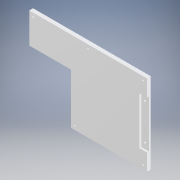
# Autodesk Inventor part: SP001b
Saved by Autodesk Inventor 2017 SP1 (Build 210196100, 196)
## iProperties
Created: 2018-01-11
Part Number: SP001b
Material: ABS Plastic
Document SubType Name: Modeling
Designer: Zach
Density: 1.06 g/cm^3
Appearance: CR White
Author: Zach
Autodesk Inventor part; units mm, degrees
ref_plane "YZ Plane" through (0, 0, 0) normal (1, 0, 0) x (0, 1, 0)
ref_plane "XZ Plane" through (0, 0, 0) normal (0, 1, 0) x (-1, 0, 0)
ref_plane "XY Plane" through (0, 0, 0) normal (0, 0, 1) x (1, 0, 0)
sketch "Sketch1" plane through (0, 0, 0) normal (0, 0, 1) x (1, 0, 0)
  line L0 (0, 0) -> (620, 0)
  line L1 (110, -213) -> (510, -213)
  line L2 (510, -213) -> (510, -80)
  line L3 (510, -80) -> (620, -80)
  line L4 (620, -80) -> (620, 0)
  line L5 (110, -213) -> (110, -80)
  line L6 (0, -80) -> (0, 0)
  line L7 (0, -80) -> (110, -80)
  point P0 (310, -213)
  point P1 (310, 0)
  dimension "d0" = 620
  dimension "d1" = 213
  dimension "d2" = 400
  dimension "d3" = 133
  constraints: 16 end point, 3 perpendicular, 2 horizontal, 2 midpoint, 2 parallel, 2 point on line, 1 vertical, 1 vertical alignment
  measures "d0" distance of L0.start L0.end
  measures "d1" distance between parallel lines of L0 L1
  measures "d2" distance of L1.start L1.end
  measures "d3" distance of L1.end L2.end
extrude "Extrusion1" add sketch "Sketch1" along normal blind 10
sketch "Sketch2" plane through (0, 0, 10) normal (0, 0, 1) x (1, 0, 0)
  line L0 (620, 0) -> (0, 0) projected
  line L1 (510, -213) -> (110, -213) projected
  line L2 (620, 0) -> (310, 0)
  line L3 (310, 0) -> (310, -213)
  line L4 (310, -213) -> (620, -213)
  line L5 (620, -213) -> (620, 0)
  constraints: 8 end point, 2 parallel, 1 horizontal, 1 midpoint, 1 perpendicular
extrude "Extrusion2" cut sketch "Sketch2" against normal through all
sketch "Sketch3" plane through (0, 0, 10) normal (0, 0, 1) x (1, 0, 0)
  circle A0 centre (10, -10) radius 2
  line L0 (310, 0) -> (0, 0) projected
  line L1 (0, 0) -> (0, -80) projected
  circle A1 centre (155, -10) radius 2
  circle A2 centre (300, -10) radius 2
  line L2 (310, -213) -> (310, 0) projected
  line L3 (10, -10) -> (300, -10) construction
  circle A3 centre (120, -203) radius 2
  line L4 (110, -80) -> (110, -213) projected
  line L5 (110, -213) -> (310, -213) projected
  circle A4 centre (300, -203) radius 2
  dimension "d8" = 4
  dimension "d9" = 10
  dimension "d10" = 10
  dimension "d11" = 4
  dimension "d12" = 4
  dimension "d13" = 10
  dimension "d14" = 4
  dimension "d15" = 10
  dimension "d16" = 10
  dimension "d17" = 4
  dimension "d18" = 10
  dimension "d19" = 10
  constraints: 5 centre point, 2 end point, 2 horizontal alignment, 1 coincident, 1 horizontal, 1 midpoint
  measures "d8" diameter of A0
  measures "d9" distance from line of L0 L3.start
  measures "d10" distance from line of L1 L3.start
  measures "d11" diameter of A1
  measures "d12" diameter of A2
  measures "d13" distance from line of L2 L3.end
  measures "d14" diameter of A3
  measures "d15" distance from line of L4 A3.centre
  measures "d16" distance from line of L5 A3.centre
  measures "d17" diameter of A4
  measures "d18" distance from line of L2 A4.centre
  measures "d19" distance from line of L5 A4.centre
extrude "Extrusion3" cut sketch "Sketch3" against normal through all
sketch "Sketch6" plane through (0, 0, 10) normal (0, 0, 1) x (1, 0, 0)
  line L0 (310, -44) -> (290, -44)
  line L1 (290, -44) -> (290, -169)
  line L2 (290, -169) -> (310, -169)
  line L3 (310, -169) -> (310, -44)
  line L4 (310, -213) -> (310, 0) projected
  point P0 (0, 0)
  point P1 (310, -106.5)
  dimension "d42" = 20
  dimension "d43" = 125
  constraints: 8 end point, 2 midpoint, 2 parallel, 1 horizontal, 1 perpendicular
  measures "d42" distance of L2.end L1.end
  measures "d43" distance of L1.end L0.end
extrude "Extrusion6" cut sketch "Sketch6" against normal blind 5
sketch "Sketch7" plane through (0, 0, 5) normal (0, 0, 1) x (1, 0, 0)
  line L0 (300, -59) -> (300, -154) construction
  circle A0 centre (300, -59) radius 2.5
  circle A1 centre (300, -154) radius 2.5
  line L1 (310, -44) -> (310, -169) projected
  point P0 (0, 0)
  point P1 (300, -106.5)
  point P2 (310, -106.5)
  dimension "d46" = 5
  dimension "d47" = 5
  dimension "d48" = 10
  dimension "d49" = 95
  constraints: 2 centre point, 2 coincident, 2 end point, 2 midpoint, 1 horizontal alignment, 1 vertical
  measures "d46" diameter of A0
  measures "d47" diameter of A1
  measures "d48" distance between parallel lines of L1 L0
  measures "d49" distance of L0.start L0.end
extrude "Extrusion7" cut sketch "Sketch7" against normal through all
body "Solid1"
